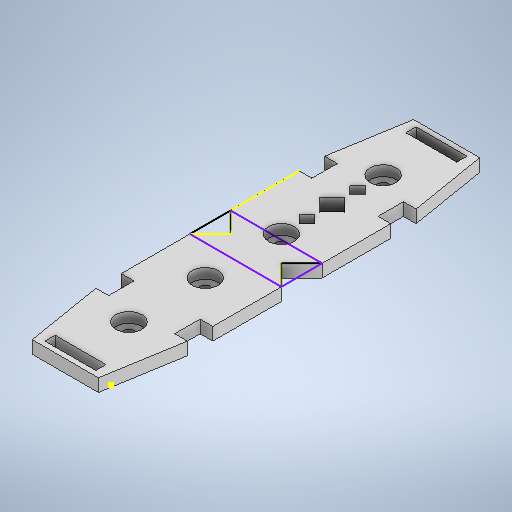
# Autodesk Inventor part: Side
Saved by Autodesk Inventor 2025.2 (Build 292293000, 293)
## iProperties
Created: 2025-04-09
Part Number: Side
Material: Generic
Document SubType Name: Modeling
Designer: 1khanhan2
Density: 1 g/cm^3
Appearance: Default
Author: 1khanhan2
Autodesk Inventor part; units mm, degrees
ref_plane "YZ Plane" through (0, 0, 0) normal (1, 0, 0) x (0, 1, 0)
ref_plane "XZ Plane" through (0, 0, 0) normal (0, 1, 0) x (-1, 0, 0)
ref_plane "XY Plane" through (0, 0, 0) normal (0, 0, 1) x (1, 0, 0)
sketch "Sketch1" plane through (0, 0, 0) normal (0, 1, 0) x (-1, 0, 0)
  line L0 (5, 0) -> (31, 0)
  line L1 (36, -30) -> (36, -120)
  line L2 (31, -150) -> (5, -150)
  line L3 (0, -120) -> (0, -30)
  circle A0 centre (18, -25) radius 5.1
  circle A1 centre (18, -55) radius 5.1
  circle A2 centre (18, -85) radius 5.1
  circle A3 centre (18, -125) radius 5.1
  line L4 (36, -30) -> (31, -30)
  line L5 (31, -30) -> (31, -40)
  line L6 (31, -40) -> (36, -40)
  line L7 (36, -120) -> (31, -120)
  line L8 (31, -120) -> (31, -110)
  line L9 (31, -110) -> (36, -110)
  line L10 (0, -30) -> (5, -30)
  line L11 (5, -30) -> (5, -40)
  line L12 (5, -40) -> (0, -40)
  line L13 (0, -120) -> (5, -120)
  line L14 (5, -120) -> (5, -110)
  line L15 (0, -110) -> (5, -110)
  circle A4 centre (18, -25) radius 2.25
  circle A5 centre (18, -55) radius 2.25
  circle A6 centre (18, -85) radius 2.25
  circle A7 centre (18, -125) radius 2.25
  line L16 (5, 0) -> (0, -30)
  line L17 (31, -150) -> (36, -120)
  line L18 (5, -150) -> (0, -120)
  line L19 (31, 0) -> (36, -30)
  line L20 (18, -100) -> (13, -105)
  line L21 (13, -105) -> (18, -110)
  line L22 (23, -105) -> (18, -110)
  line L23 (23, -105) -> (18, -100)
  line L24 (21, -114.95) -> (18, -117.95)
  line L25 (15, -114.95) -> (18, -117.95)
  line L26 (15, -114.95) -> (18, -111.95)
  line L27 (18, -111.95) -> (21, -114.95)
  line L28 (21, -95.05) -> (18, -98.05)
  line L29 (18, -98.05) -> (15, -95.05)
  line L30 (15, -95.05) -> (18, -92.05)
  line L31 (18, -92.05) -> (21, -95.05)
  line L32 (31, -150) -> (28, -150)
  line L33 (5, -150) -> (8, -150)
  line L34 (8, -148) -> (28, -148)
  line L35 (8, -148) -> (8, -144)
  line L36 (8, -144) -> (28, -144)
  line L37 (28, -144) -> (28, -148)
  line L38 (31, 0) -> (28, 0)
  line L39 (5, 0) -> (8, 0)
  line L40 (8, -2) -> (28, -2)
  line L41 (28, -2) -> (28, -6)
  line L42 (28, -6) -> (8, -6)
  line L43 (8, -6) -> (8, -2)
  line L44 (36, -75) -> (36, -83)
  line L45 (36, -75) -> (36, -67)
  line L46 (36, -67) -> (28, -75)
  line L47 (36, -83) -> (28, -75)
  line L48 (0, -75) -> (0, -83)
  line L49 (0, -75) -> (0, -67)
  line L50 (0, -67) -> (8, -75)
  line L51 (0, -83) -> (8, -75)
  point P0 (0, 0)
  point P1 (18, 0)
  point P2 (18, -150)
  dimension "d2" = 10.2
  dimension "d3" = 25
  dimension "d4" = 10.2
  dimension "d5" = 30
  dimension "d6" = 10.2
  dimension "d7" = 30
  dimension "d8" = 10.2
  dimension "d9" = 40
  dimension "d10" = 25
  dimension "d12" = 5
  dimension "d13" = 10
  dimension "d15" = 10
  dimension "d17" = 5
  dimension "d19" = 5
  dimension "d22" = 4.5
  dimension "d23" = 4.5
  dimension "d24" = 4.5
  dimension "d25" = 4.5
  dimension "d38" = 3
  dimension "d39" = 2
  dimension "d41" = 2
  dimension "d42" = 4
  dimension "d44" = 2
  dimension "d45" = 3
  dimension "d46" = 4
  dimension "d50" = 8
  dimension "d51" = 8
  constraints: 104 end point, 17 perpendicular, 16 point on line, 8 centre point, 4 coincident, 4 midpoint, 4 parallel, 1 horizontal
  measures "d2" diameter of A0
  measures "d3" distance of A0.centre point (18, 0)
  measures "d4" diameter of A1
  measures "d5" distance of A1.centre A0.centre
  measures "d6" diameter of A2
  measures "d7" distance of A2.centre A1.centre
  measures "d8" diameter of A3
  measures "d9" distance of A3.centre A2.centre
  measures "d10" distance of point (18, -150) A3.centre
  measures "d12" distance of L1.start L4.end
  measures "d13" distance of L4.end L5.end
  measures "d15" distance of L7.end L8.end
  measures "d17" distance of L3.end L10.end
  measures "d19" distance of L3.start L13.end
  measures "d22" diameter of A4
  measures "d23" diameter of A5
  measures "d24" diameter of A6
  measures "d25" diameter of A7
  measures "d38" distance of L2.start L32.end
  measures "d39" distance of L32.end L34.end
  measures "d41" distance of L33.end L34.start
  measures "d42" distance of L34.start L35.end
  measures "d44" distance of L38.end L40.end
  measures "d45" distance of L0.start L39.end
  measures "d46" distance of L40.end L41.end
  measures "d50" distance of L48.start L48.end
  measures "d51" distance of L48.start L49.end
extrude "Extrusion1" add sketch "Sketch1" along normal blind 5 contours L0 L19 L4 L5 L6 L1 L46 L47 L9 L8 L7 L17 L2 L18 L13 L14 L15 L3 L51 L50 L12 L11 L10 L16
extrude "Extrusion2" add sketch "Sketch1" along normal blind 1 contours A0 | A1 | A2 | A3
sketch "Sketch2" plane through (0, 5, 0) normal (0, 1, 0) x (1, 0, 0)
  line L0 (-28, 75) -> (-36, 67) projected
  line L1 (-36, 110) -> (-36, 83) projected
  line L2 (-36, 67) -> (-36, 83)
  line L3 (-36, 83) -> (-28, 75) projected
  line L4 (-36, 83) -> (-28, 75)
  line L5 (-28, 75) -> (-36, 67)
  line L6 (0, 67) -> (-8, 75) projected
  line L7 (-8, 75) -> (0, 67)
  line L8 (0, 67) -> (0, 83)
  line L9 (0, 83) -> (-8, 75)
  line L10 (-36, 67) -> (0, 67)
  line L11 (-36, 83) -> (0, 83)
  point P0 (0, 0)
  constraints: 16 end point, 3 equal length, 2 perpendicular, 1 vertical
body "Solid1"
